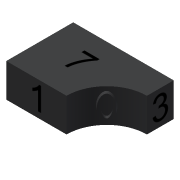
# Autodesk Inventor part: block
Saved by Autodesk Inventor 2022 Beta2 (Build 260130000, 130) ContinuousBuild 0
## iProperties
Shininess: 64.0
Length Units: 11269
Angle Units: 11279
Time Units: 11290
Mass Units: 11283
Length Display Precision: 3
Angle Display Precision: 2
Compacted: True
Part Number: block
Document SubType Name: Modeling
Created: 2004-04-21
Designer: mpaknia
Manufacturer: Standard
Standards Organization: Custom
Density: 1 g/cm^3
Material: Generic
Appearance: Generic
Density: 0.0
Volumn: 0.0
Area: 0.0
PropertySet Name: Model Information
Control State: 0
Master: False
Checked Out: False
Author: mpaknia
Autodesk Inventor part; units mm, degrees
ref_plane "YZ Plane" through (0, 0, 0) normal (1, 0, 0) x (0, 1, 0)
ref_plane "XZ Plane" through (0, 0, 0) normal (0, 1, 0) x (-1, 0, 0)
sketch "Sketch1" plane through (0, 0, 0) normal (0, 0, 1) x (1, 0, 0)
  line L0 (0, 0) -> (18, 0)
  line L1 (30, 12) -> (30, 20)
  line L2 (30, 20) -> (0, 20)
  line L3 (0, 20) -> (0, 0)
  arc A0 (30, 12) -> (18, 0) centre (30, 0) ccw
  dimension "d0" = 30
  dimension "d1" = 20
  dimension "d2" = 12
  constraints: 8 end point, 2 parallel, 2 point on circle, 1 centre point, 1 horizontal, 1 horizontal alignment, 1 perpendicular, 1 vertical alignment
  measures "d0" distance between parallel lines of L1 L3
  measures "d1" distance between parallel lines of L0 L2
  measures "d2" radius of A0
extrude "Extrusion1" add sketch "Sketch1" along normal blind 10
sketch "Sketch2" plane through (0, 0, 0) normal (0, -1, 0) x (1, 0, 0)
  line L0 (6.7288, 8.7537) -> (12.1656, 8.7537) construction
  line L1 (12.1656, 8.7537) -> (12.1656, 1.727) construction
  line L2 (12.1656, 1.727) -> (6.7288, 1.727) construction
  line L3 (6.7288, 1.727) -> (6.7288, 8.7537) construction
  constraints: 2 other
sketch "Sketch3" plane through (30, 12, 0) normal (1, 0, 0) x (0, 0, -1)
  line L0 (-8.6261, 1.3146) -> (-8.6261, 6.7514) construction
  line L1 (-8.6261, 6.7514) -> (-1.482, 6.7514) construction
  line L2 (-1.482, 6.7514) -> (-1.482, 1.3146) construction
  line L3 (-1.482, 1.3146) -> (-8.6261, 1.3146) construction
  constraints: 2 other
sketch "Sketch4" plane through (0, 20, 0) normal (0, 1, 0) x (1, 0, 0)
  line L0 (16.9923, -8.3919) -> (11.5555, -8.3919) construction
  line L1 (11.5555, -8.3919) -> (11.5555, -1.3919) construction
  line L2 (11.5555, -1.3919) -> (16.9923, -1.3919) construction
  line L3 (16.9923, -1.3919) -> (16.9923, -8.3919) construction
  constraints: 2 other
sketch "Sketch5" plane through (0, 0, 0) normal (-1, 0, 0) x (0, 0, 1)
  line L0 (8.5269, 13.0876) -> (8.5269, 7.6509) construction
  line L1 (8.5269, 7.6509) -> (1.5002, 7.6509) construction
  line L2 (1.5002, 7.6509) -> (1.5002, 13.0876) construction
  line L3 (1.5002, 13.0876) -> (8.5269, 13.0876) construction
  constraints: 2 other
sketch "Sketch6" plane through (0, 0, 10) normal (0, 0, 1) x (1, 0, 0)
  line L0 (8.4775, 14.4017) -> (13.9142, 14.4017) construction
  line L1 (13.9142, 14.4017) -> (13.9142, 7.4924) construction
  line L2 (13.9142, 7.4924) -> (8.4775, 7.4924) construction
  line L3 (8.4775, 7.4924) -> (8.4775, 14.4017) construction
  constraints: 2 other
sketch "Sketch7" plane through (0, 0, 0) normal (0, 0, -1) x (-1, 0, 0)
  line L0 (-16.3171, 15.4982) -> (-10.8803, 15.4982) construction
  line L1 (-10.8803, 15.4982) -> (-10.8803, 8.3541) construction
  line L2 (-10.8803, 8.3541) -> (-16.3171, 8.3541) construction
  line L3 (-16.3171, 8.3541) -> (-16.3171, 15.4982) construction
  constraints: 2 other
ref_plane "Work Plane1" through (18, 0, 0) normal (-0.7071068, 0.7071068, 0) x (0, 0, 1)
sketch "Sketch9" plane through (18, 0, 0) normal (-0.7071068, 0.7071068, 0) x (0, 0, 1)
  line L0 (8.7931, 11.1492) -> (8.7931, 5.7124) construction
  line L1 (8.7931, 5.7124) -> (1.7665, 5.7124) construction
  line L2 (1.7665, 5.7124) -> (1.7665, 11.1492) construction
  line L3 (1.7665, 11.1492) -> (8.7931, 11.1492) construction
  spline S0 degree 4 poles (5.2185, 10.7437) (6.4616, 10.7437) (7.9768, 10.2315) (8.7931, 9.2284) (8.7931, 8.4601) knots 0 0 0 0 0 1 1 1 1 1
  spline S1 degree 5 poles (8.7931, 8.4601) (8.7931, 7.8999) (8.3396, 7.0463) (7.486, 6.4967) (6.2589, 6.1819) (5.2185, 6.1819) knots 0 0 0 0 0 0 1 1 1 1 1 1
  spline S2 degree 4 poles (5.2185, 6.1819) (3.986, 6.1819) (2.4707, 6.6888) (1.6491, 7.6972) (1.6491, 8.4601) knots 0 0 0 0 0 1 1 1 1 1
  spline S3 degree 2 poles (1.6491, 8.4601) (1.6491, 9.4739) (2.3694, 10.0501) knots 0 0 0 1 1 1
  spline S4 degree 2 poles (2.3694, 10.0501) (3.2497, 10.7437) (5.2185, 10.7437) knots 0 0 0 1 1 1
  spline S5 degree 3 poles (5.2185, 9.858) (3.4898, 9.858) (2.3534, 9.0524) (2.3534, 8.4601) knots 0 0 0 0 1 1 1 1
  spline S6 degree 3 poles (2.3534, 8.4601) (2.3534, 7.8733) (3.4951, 7.0676) (5.2185, 7.0676) knots 0 0 0 0 1 1 1 1
  spline S7 degree 3 poles (5.2185, 7.0676) (6.9471, 7.0676) (8.0835, 7.8733) (8.0835, 8.4708) knots 0 0 0 0 1 1 1 1
  spline S8 degree 2 poles (8.0835, 8.4708) (8.0835, 9.063) (7.582, 9.4152) knots 0 0 0 1 1 1
  spline S9 degree 2 poles (7.582, 9.4152) (6.9418, 9.858) (5.2185, 9.858) knots 0 0 0 1 1 1
  constraints: 2 other
emboss "Emboss1" sketch "Sketch9" operation add depth 1 direction (0.7071068, -0.7071068, 0) wrap yes faces at (21.8379, 8.7966, 6.6667)
body "Solid1"
